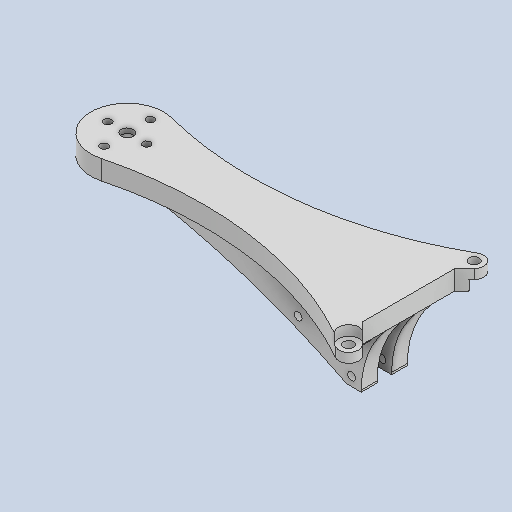
# Autodesk Inventor part: brat
Saved by Autodesk Inventor 2025.2 (Build 292293000, 293)
## iProperties
Created: 2025-03-18
Part Number: brat
Material: Generic
Document SubType Name: Modeling
Designer: mirewn
Density: 1 g/cm^3
Appearance: Default
Author: mirewn
Autodesk Inventor part; units mm, degrees
ref_plane "YZ Plane" through (0, 0, 0) normal (1, 0, 0) x (0, 1, 0)
ref_plane "XZ Plane" through (0, 0, 0) normal (0, 1, 0) x (-1, 0, 0)
ref_plane "XY Plane" through (0, 0, 0) normal (0, 0, 1) x (1, 0, 0)
sketch "Sketch1" plane through (0, 0, 0) normal (0, 1, 0) x (-1, 0, 0)
  line L0 (0, 0) -> (105.9629, 0) construction
  line L1 (105.9629, 0) -> (105.9629, -9.5) construction
  circle A0 centre (105.9629, -9.5) radius 1.6
  circle A1 centre (113.9629, 0) radius 1.6
  circle A2 centre (105.9629, -9.5) radius 1.6
  circle A3 centre (97.9629, 0) radius 1.6
  circle A4 centre (105.9629, 9.5) radius 1.6
  circle A5 centre (105.9629, 0) radius 15
  circle A6 centre (105.9629, 0) radius 2.5
  line L2 (3, -40) -> (-37, 0) construction
  line L3 (-7.5, -16.5) -> (-14, -23)
  circle A7 centre (-11.1716, -25.8284) radius 4
  circle A8 centre (-11.1716, -25.8284) radius 2.1
  arc A9 (102.2211, -14.5258) -> (-9.1982, -29.3078) centre (64.8022, -159.7836) ccw
  line L4 (3, 40) -> (-37, 0) construction
  line L5 (-7.5, 16.5) -> (-14, 23)
  circle A10 centre (-11.1716, 25.8284) radius 4
  circle A11 centre (-11.1716, 25.8284) radius 2.1
  arc A12 (-9.1982, 29.3078) -> (102.2211, 14.5258) centre (64.8022, 159.7836) ccw
  line L6 (-10, 19) -> (-10, -19)
  arc A13 (-12.9845, 21.9845) -> (-6.9989, 26.6354) centre (-11.1716, 25.8284) ccw
  arc A14 (-7.9621, -28.6144) -> (-12.9845, -21.9845) centre (-11.1716, -25.8284) ccw
  arc A15 (-6.9989, 26.6354) -> (-7.9621, 28.6144) centre (-11.1716, 25.8284) ccw
  point P0 (-16.1526, 27.519)
  point P1 (-14, -23)
  point P2 (102.2211, 14.5258)
  point P3 (-14, 23)
  point P4 (-10, 0)
  point P5 (-12.9845, -21.9845)
  dimension "d5" = 30
  dimension "d67" = 8
  dimension "d1" = 9.5
  dimension "d2" = 3.2
  dimension "d3" = 3.2
  dimension "d4" = 8
  dimension "d55" = 5
  dimension "d68" = 4
  dimension "d69" = 4.2
  dimension "d70" = 150
  dimension "d82" = 10
  dimension "d84" = 38
  dimension "d85" = 105.963
  dimension "d86" = 4.25
  constraints: 14 end point, 13 centre point, 13 symmetric about line, 11 point on circle, 8 point on line, 6 coincident, 2 horizontal, 2 vertical, 1 horizontal alignment, 1 midpoint, 1 perpendicular, 18 other
  measures "d1" distance of L0.end L1.end
  measures "d2" diameter of A0
  measures "d3" diameter of A1
  measures "d4" distance of L0.end A1.centre
  measures "d55" diameter of A6
  measures "d68" distance of L3.end point (-11.172, -25.828)
  measures "d69" diameter of A8
  measures "d70" radius of A9
  measures "d82" distance of point (-10, 0) L0.start
  measures "d84" distance of L6.start L6.end
  measures "d85" distance of L0.end L0.start
  measures "d86" radius of A13
extrude "Extrusion1" add sketch "Sketch1" along normal blind 8 contours A5 | A5 A9 A14 L3 L6 L5 A13 A15 A12 | A6
extrude "Extrusion2" add sketch "Sketch1" along normal blind 3.9 contours A15 A13 L5 A10 A12 | A10
extrude "Extrusion3" add sketch "Sketch1" against normal blind 3.9 from surface at 8 contours A9 A7 L3 A14 | A7
extrude "Extrusion9" cut sketch "Sketch1" against normal blind 2 from surface at 8 contours A6
sketch "Sketch2" plane through (0, 0, 0) normal (0, 0, 1) x (1, 0, 0)
  line L0 (0, 0) -> (-3, 0) projected
  line L1 (0, 0) -> (0, -30)
  line L2 (-98.8932, 0) -> (-6, 0) projected
  arc A0 (0, -30) -> (-85, 0) centre (-137.8451, -285.1445) ccw
  line L3 (-6, -26.8484) -> (0, -26.8484)
  line L4 (0, 0) -> (-85, 0)
  line L5 (0, -23.1484) -> (-13.5147, -23.1484) construction
  circle A1 centre (-4, -23.1484) radius 1.6
  arc A2 (10, 0) -> (0, -26.8484) centre (39.9981, -26.4597) ccw
  line L6 (10, 0) -> (0, 0)
  line L7 (12.9845, 8) -> (10, 8) projected
  point P0 (0, -15)
  point P1 (-3, 0)
  point P2 (-6, 0)
  point P3 (-85, 0)
  point P4 (12.622, 8)
  point P5 (0, 8)
  point P6 (0, -26.0709)
  point P7 (14, 8)
  point P8 (12.7592, 8)
  dimension "d16" = 290
  dimension "d17" = 85
  dimension "d18" = 6
  dimension "d19" = 30
  dimension "d63" = 3.7
  dimension "d64" = 3.2
  dimension "d65" = 4
  dimension "d79" = 10
  dimension "d80" = 40
  constraints: 10 end point, 6 point on circle, 5 point on line, 3 centre point, 1 coincident, 1 collinear, 1 midpoint, 1 parallel, 1 perpendicular, 1 vertical
  measures "d16" radius of A0
  measures "d17" horizontal distance of point (0, -15) L4.end
  measures "d18" distance of L3.start L3.end
  measures "d19" distance of L1.end L0.start
  measures "d63" distance between parallel lines of L3 L5
  measures "d64" diameter of A1
  measures "d65" distance from line of L1 A1.centre
  measures "d79" distance from line of L6.start L1
  measures "d80" radius of A2
extrude "Extrusion4" add sketch "Sketch2" along normal mid plane 19 contours L6 A2 L3 A0 L2 L4 L0
extrude "Extrusion11" cut sketch "Sketch2" along normal mid plane 6 contours L6 A2 L3 A0 L2 L4 L0 | A1
sketch "Sketch9" plane through (0, 0, 9.5) normal (0, 0, 1) x (1, 0, 0)
  circle A0 centre (-26, -12.7093) radius 1.6
  arc A1 (-6, -26.8484) -> (-85, 0) centre (-137.8451, -285.1445) ccw projected
  line L0 (0, -26.8484) -> (0, 0) projected
  line L1 (-137.8451, -285.1445) -> (-26, -12.7093) construction
  line L2 (-26, -12.7093) -> (-21.4388, -1.5991) construction
  circle A2 centre (-23.5314, -6.6963) radius 1.6
  line L3 (0, 0) -> (0, -45) construction
  point P0 (0, -13.4242)
  dimension "d71" = 3.2
  dimension "d72" = 294.5
  dimension "d73" = 26
  dimension "d75" = 3.2
  dimension "d76" = 6.5
  constraints: 6 end point, 3 point on line, 2 centre point, 1 midpoint
  measures "d71" diameter of A0
  measures "d72" distance of L1.start L1.end
  measures "d73" horizontal distance of point (0, -13.424) L1.end
  measures "d75" diameter of A2
  measures "d76" distance of L1.end A2.centre
extrude "Extrusion12" cut sketch "Sketch9" against normal through all
sketch "Sketch10" plane through (10, 0, -19) normal (1, 0, 0) x (0, 0, -1)
  line L0 (-38, 0) -> (-28.5, 0) projected
  line L1 (-28.5, 0) -> (-28.5, -7)
  line L2 (-28.5, -26.8484) -> (-28.5, 0) projected
  line L3 (-28.5, 0) -> (-37.25, 0)
  circle A0 centre (-31.1, -2.6) radius 2.6
  arc A1 (-34.85, -2.6) -> (-31.1, -6.35) centre (-31.1, -2.6) ccw
  line L4 (-34.85, -2.6) -> (-34.85, 0)
  line L5 (-31.1, -6.35) -> (-28.5, -6.35)
  line L6 (-31.1, -5.2) -> (-28.5, -5.2)
  line L7 (-33.7, -2.6) -> (-33.7, 0)
  arc A2 (-28.5, -5.3023) -> (-33.8023, 0) centre (-31.1, -2.6) ccw
  arc A3 (-31.1, -6.35) -> (-28.5, -5.3023) centre (-31.1, -2.6) ccw construction
  point P0 (-19, 0)
  point P1 (-33.7, 0)
  point P2 (-34.85, 0)
  point P3 (-32.4068, -0.3523)
  point P4 (-31.1, 0)
  point P5 (-28.5, -2.6)
  point P6 (-31.1, 0)
  dimension "d101" = 5.2
  dimension "d102" = 7.5
  constraints: 12 end point, 10 tangent, 9 point on circle, 7 point on line, 5 perpendicular, 4 centre point, 1 coincident
  measures "d101" diameter of A0
  measures "d102" diameter of A1
extrude "Extrusion16" add sketch "Sketch10" against normal blind 25 contours L0 L7 A0 L6 L1 L5 A1 L4
extrude "Extrusion17" cut sketch "Sketch10" against normal blind 21 contours L0 L7 A0 L6 L1 L5 A1 L4 | L0 A0 L7 | L0 L1 A0 | L6 A0 L1
extrude "Extrusion18" add sketch "Sketch10" against normal blind 10 contours L0 L7 A0 L6 L1 L5 A1 L4
extrude "Extrusion19" cut sketch "Sketch10" against normal blind 6 contours L0 L7 A0 L6 L1 L5 A1 L4 | L0 A0 L7 | L0 L1 A0 | L6 A0 L1
chamfer "Chamfer1" distance 1.5 angle 45 4 edges at (-104.3629, 0, 9.5) (-96.3629, 0, 0) (-112.3629, 0, 0) (-104.3629, 0, -9.5)
body "Solid1"
